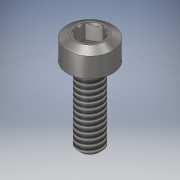
# Autodesk Inventor part: Bolt_M1.6x0.35_5mm_SH
Saved by Autodesk Inventor 2018 (Build 220112000, 112)
## iProperties
Manager: Bradley
Company: Zetta & Zepto Technology
Created: 2016-07-03
Part Number: Bolt_M1.6x0.35_5mm_SH
Material: Stainless Steel
Document SubType Name: Modeling
Designer: Bradley
Density: 8 g/cm^3
Appearance: Semi-Polished
Description: SCM4006-3H3
Stock Number: 80110
Author: Bradley
Autodesk Inventor part; units mm, degrees
ref_plane "YZ Plane" through (0, 0, 0) normal (1, 0, 0) x (0, 1, 0)
ref_plane "XZ Plane" through (0, 0, 0) normal (0, 1, 0) x (-1, 0, 0)
ref_plane "XY Plane" through (0, 0, 0) normal (0, 0, 1) x (1, 0, 0)
sketch "Sketch1" plane through (0, 0, 0) normal (0, 0, 1) x (1, 0, 0)
  line L0 (0, 3.3) -> (0, -3.3)
  line L1 (0, -3.3) -> (0.6, -3.3)
  line L2 (0.6, -3.3) -> (0.8, -3.1)
  line L3 (0.8, -3.1) -> (0.8, 1.6)
  line L4 (0.9, 1.7) -> (1.5, 1.7)
  line L5 (1.5, 1.7) -> (1.5, 3.0113)
  line L6 (1, 3.3) -> (0, 3.3)
  arc A0 (0.9, 1.7) -> (0.8, 1.6) centre (0.9, 1.6) ccw
  line L7 (1, 3.3) -> (1.5, 3.0113)
  point P0 (0, 0)
  point P1 (1.5, 3.3)
  point P2 (0, 0)
  dimension "d0" = 3
  dimension "d1" = 1.6
  dimension "d3" = 1.6
  dimension "d4" = 1.8
  dimension "d5" = 135
  dimension "d6" = 0.2
  dimension "d7" = 5
  dimension "d9" = 0.5
  dimension "d10" = 30
  constraints: 16 end point, 4 perpendicular, 2 point on circle, 2 point on line, 2 tangent, 1 centre point, 1 coincident, 1 midpoint, 1 parallel, 1 vertical
  measures "d0" diameter of L5 L0
  measures "d1" distance of L4.end point (1.5, 3.3)
  measures "d3" diameter of L3 L0
  measures "d4" diameter of L4.start L0
  measures "d5" angle of L3 L2
  measures "d6" horizontal distance of L1.end L2.end
  measures "d7" distance between parallel lines of L1 L4
  measures "d9" distance of L6.start point (1.5, 3.3)
  measures "d10" angle of L6 L7
revolve "Revolution1" add sketch "Sketch1" angle 360 about axis through (0, 3.3, 0) along (0, -1, 0)
sketch "Sketch2" plane through (0, 3.3, 0) normal (0, 1, 0) x (1, 0, 0)
  line L0 (0, -0.866) -> (-0.75, -0.433)
  line L1 (-0.75, -0.433) -> (-0.75, 0.433)
  line L2 (-0.75, 0.433) -> (0, 0.866)
  line L3 (0, 0.866) -> (0.75, 0.433)
  line L4 (0.75, 0.433) -> (0.75, -0.433)
  line L5 (0.75, -0.433) -> (0, -0.866)
  point P0 (0, 0)
  point P1 (0, 0)
  dimension "d11" = 1.5
  constraints: 12 end point, 1 coincident, 1 vertical, 13 other
  measures "d11" distance between parallel lines of L4 L1
extrude "Extrusion1" cut sketch "Sketch2" against normal blind 1
thread "Thread1" size "M1.6x0.35" class "6g" standard "ANSI Metric M Profile" full length
sketch "Sketch3" plane through (0, 0, 0) normal (1, 0, 0) x (0, 1, 0)
  line L0 (3.3, 0.866) -> (2.8, 0.366)
  line L1 (2.8, 0.366) -> (3.3, 0.366)
  line L2 (3.3, 0.866) -> (3.3, 0.366)
  line L3 (-0.66, 0) -> (3.96, 0) projected
  point P0 (0, 0)
  dimension "d16" = 0.5
  constraints: 6 end point, 1 horizontal, 1 perpendicular, 1 vertical
  measures "d16" distance of L0.start L1.end
revolve "Revolution2" cut sketch "Sketch3" angle 360 about axis through (0, -10, 0) along (0, 1, 0)
body "Solid1"
